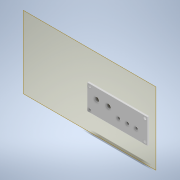
# Autodesk Inventor part: InterfacePlate
Saved by Autodesk Inventor 2022.2 (Build 262287000, 287)
## iProperties
Created: 2022-01-15
Part Number: InterfacePlate
Material: Generic
Document SubType Name: Modeling
Designer: siwat
Density: 1 g/cm^3
Appearance: Default
Author: siwat
Autodesk Inventor part; units mm, degrees
ref_plane "YZ Plane" through (0, 0, 0) normal (1, 0, 0) x (0, 1, 0)
ref_plane "XZ Plane" through (0, 0, 0) normal (0, 1, 0) x (-1, 0, 0)
ref_plane "XY Plane" through (0, 0, 0) normal (0, 0, 1) x (1, 0, 0)
ref_plane "Work Plane1" through (0, 0, 0) normal (0, 0, 1) x (1, 0, 0)
sketch "Sketch1" plane through (0, 0, 0) normal (0, 0, 1) x (1, 0, 0)
  line L0 (67.7271, 45.3897) -> (135.6749, 45.3897)
  line L1 (135.6749, 45.3897) -> (135.6749, 17.2701)
  line L2 (135.6749, 17.2701) -> (67.7271, 17.2701)
  line L3 (67.7271, 17.2701) -> (67.7271, 45.3897)
  circle A0 centre (70.3236, 42.7621) radius 1.5
  circle A1 centre (70.2655, 19.7679) radius 1.5
  circle A2 centre (132.8977, 19.6632) radius 1.5
  circle A3 centre (132.9442, 42.6673) radius 1.5
  point P0 (0, 0)
  dimension "d0" = 3
  dimension "d1" = 3
  dimension "d2" = 3
  dimension "d3" = 3
  constraints: 8 end point, 4 centre point, 2 parallel, 1 horizontal, 1 perpendicular
  measures "d0" diameter of A0
  measures "d1" diameter of A1
  measures "d2" diameter of A2
  measures "d3" diameter of A3
extrude "Extrusion1" add sketch "Sketch1" along normal blind 2
sketch "Sketch2" plane through (0, 0, 0) normal (0, 0, -1) x (-1, 0, 0)
  line L0 (-130.7904, 21.7727) -> (-72.4709, 21.7727)
  line L1 (-72.4709, 21.7727) -> (-72.4709, 40.605)
  line L2 (-72.4709, 40.605) -> (-130.7904, 40.605)
  line L3 (-130.7904, 40.605) -> (-130.7904, 21.7727)
  point P0 (0, 0)
  constraints: 8 end point, 2 parallel, 1 horizontal, 1 perpendicular
extrude "Extrusion2" add sketch "Sketch2" along normal blind 3
sketch "Sketch3" plane through (0, 0, -3) normal (0, 0, -1) x (-1, 0, 0)
  circle A0 centre (-123.1484, 27.6797) radius 1.75
  line L0 (-121.6186, 32.121) -> (-111.2555, 32.121)
  circle A1 centre (-113.1484, 27.6797) radius 1.75
  circle A2 centre (-103.1484, 27.6797) radius 1.75
  circle A3 centre (-91.5974, 33.7589) radius 2.5
  circle A4 centre (-78.3445, 33.7589) radius 2.5
  point P0 (0, 0)
  dimension "d8" = 3.5
  dimension "d11" = 10
  dimension "d16" = 5
  dimension "d17" = 5
  constraints: 5 centre point, 2 end point, 2 horizontal, 4 other
  measures "d8" diameter of A0
  measures "d11" distance of A0.centre A1.centre
  measures "d16" diameter of A3
  measures "d17" diameter of A4
extrude "Extrusion3" cut sketch "Sketch3" against normal up to surface (5 mm away)
sketch "Sketch4" plane through (0, 0, -3) normal (0, 0, -1) x (-1, 0, 0)
  line L0 (-126.3413, 33.4304) -> (-118.9387, 33.4304) construction
  line L1 (-118.9387, 33.4304) -> (-118.9387, 30.3319) construction
  line L2 (-118.9387, 30.3319) -> (-126.3413, 30.3319) construction
  line L3 (-126.3413, 30.3319) -> (-126.3413, 33.4304) construction
  line L4 (-116.3929, 33.3925) -> (-109.1583, 33.3925) construction
  line L5 (-109.1583, 33.3925) -> (-109.1583, 30.3319) construction
  line L6 (-109.1583, 30.3319) -> (-116.3929, 30.3319) construction
  line L7 (-116.3929, 30.3319) -> (-116.3929, 33.3925) construction
  line L8 (-107.7125, 33.476) -> (-98.1289, 33.476) construction
  line L9 (-98.1289, 33.476) -> (-98.1289, 30.3319) construction
  line L10 (-98.1289, 30.3319) -> (-107.7125, 30.3319) construction
  line L11 (-107.7125, 30.3319) -> (-107.7125, 33.476) construction
  line L12 (-95.4359, 29.1892) -> (-86.7439, 29.1892) construction
  line L13 (-86.7439, 29.1892) -> (-86.7439, 26.1412) construction
  line L14 (-86.7439, 26.1412) -> (-95.4359, 26.1412) construction
  line L15 (-95.4359, 26.1412) -> (-95.4359, 29.1892) construction
  line L16 (-80.7485, 29.2979) -> (-75.9197, 29.2979) construction
  line L17 (-75.9197, 29.2979) -> (-75.9197, 26.1412) construction
  line L18 (-75.9197, 26.1412) -> (-80.7485, 26.1412) construction
  line L19 (-80.7485, 26.1412) -> (-80.7485, 29.2979) construction
  line L20 (-123.6737, 30.3824) -> (-124.1998, 30.3824)
  line L21 (-124.1998, 30.3824) -> (-125.1631, 31.5952)
  line L22 (-125.1631, 31.5952) -> (-125.6275, 31.5952)
  line L23 (-125.6275, 31.5952) -> (-125.6275, 30.3824)
  line L24 (-125.6275, 30.3824) -> (-126.0326, 30.3824)
  line L25 (-126.0326, 30.3824) -> (-126.0326, 33.4304)
  line L26 (-126.0326, 33.4304) -> (-125.2471, 33.4304)
  spline S0 degree 2 poles (-125.2471, 33.4304) (-124.9853, 33.4304) (-124.6321, 33.3736) (-124.4715, 33.2699) knots 0 0 0 1 2 2 2
  spline S1 degree 2 poles (-124.4715, 33.2699) (-124.311, 33.1661) (-124.1257, 32.8426) (-124.1257, 32.603) knots 0 0 0 1 2 2 2
  spline S2 degree 2 poles (-124.1257, 32.603) (-124.1257, 32.2695) (-124.4666, 31.8175) (-124.758, 31.7088) knots 0 0 0 1 2 2 2
  line L27 (-124.758, 31.7088) -> (-123.6737, 30.3824)
  spline S3 degree 2 poles (-124.5481, 32.5709) (-124.5481, 32.7042) (-124.642, 32.9093) (-124.7408, 32.9759) knots 0 0 0 1 2 2 2
  spline S4 degree 2 poles (-124.7408, 32.9759) (-124.8272, 33.0328) (-125.0569, 33.0797) (-125.2249, 33.0797) knots 0 0 0 1 2 2 2
  line L28 (-125.2249, 33.0797) -> (-125.6275, 33.0797)
  line L29 (-125.6275, 33.0797) -> (-125.6275, 31.9336)
  line L30 (-125.6275, 31.9336) -> (-125.2718, 31.9336)
  spline S5 degree 2 poles (-125.2718, 31.9336) (-125.0964, 31.9336) (-124.8173, 31.9953) (-124.721, 32.0917) knots 0 0 0 1 2 2 2
  spline S6 degree 2 poles (-124.721, 32.0917) (-124.6321, 32.1757) (-124.5481, 32.4128) (-124.5481, 32.5709) knots 0 0 0 1 2 2 2
  line L31 (-123.4316, 30.3824) -> (-123.4316, 33.4304)
  line L32 (-123.4316, 33.4304) -> (-121.5248, 33.4304)
  line L33 (-121.5248, 33.4304) -> (-121.5248, 33.0698)
  line L34 (-121.5248, 33.0698) -> (-123.0266, 33.0698)
  line L35 (-123.0266, 33.0698) -> (-123.0266, 32.2349)
  line L36 (-123.0266, 32.2349) -> (-121.6261, 32.2349)
  line L37 (-121.6261, 32.2349) -> (-121.6261, 31.8743)
  line L38 (-121.6261, 31.8743) -> (-123.0266, 31.8743)
  line L39 (-123.0266, 31.8743) -> (-123.0266, 30.743)
  line L40 (-123.0266, 30.743) -> (-121.5248, 30.743)
  line L41 (-121.5248, 30.743) -> (-121.5248, 30.3824)
  line L42 (-121.5248, 30.3824) -> (-123.4316, 30.3824)
  line L43 (-120.3688, 30.3824) -> (-120.3688, 33.0698)
  line L44 (-120.3688, 33.0698) -> (-121.3914, 33.0698)
  line L45 (-121.3914, 33.0698) -> (-121.3914, 33.4304)
  line L46 (-121.3914, 33.4304) -> (-118.9412, 33.4304)
  line L47 (-118.9412, 33.4304) -> (-118.9412, 33.0698)
  line L48 (-118.9412, 33.0698) -> (-119.9637, 33.0698)
  line L49 (-119.9637, 33.0698) -> (-119.9637, 30.3824)
  line L50 (-119.9637, 30.3824) -> (-120.3688, 30.3824)
  line L51 (-116.0842, 30.3445) -> (-116.0842, 33.3925)
  line L52 (-116.0842, 33.3925) -> (-114.1773, 33.3925)
  line L53 (-114.1773, 33.3925) -> (-114.1773, 33.0319)
  line L54 (-114.1773, 33.0319) -> (-115.6791, 33.0319)
  line L55 (-115.6791, 33.0319) -> (-115.6791, 32.1971)
  line L56 (-115.6791, 32.1971) -> (-114.2786, 32.1971)
  line L57 (-114.2786, 32.1971) -> (-114.2786, 31.8364)
  line L58 (-114.2786, 31.8364) -> (-115.6791, 31.8364)
  line L59 (-115.6791, 31.8364) -> (-115.6791, 30.7052)
  line L60 (-115.6791, 30.7052) -> (-114.1773, 30.7052)
  line L61 (-114.1773, 30.7052) -> (-114.1773, 30.3445)
  line L62 (-114.1773, 30.3445) -> (-116.0842, 30.3445)
  line L63 (-111.6258, 30.3445) -> (-112.0902, 30.3445)
  line L64 (-112.0902, 30.3445) -> (-112.8312, 31.5598)
  line L65 (-112.8312, 31.5598) -> (-113.587, 30.3445)
  line L66 (-113.587, 30.3445) -> (-114.0242, 30.3445)
  line L67 (-114.0242, 30.3445) -> (-113.0535, 31.871)
  line L68 (-113.0535, 31.871) -> (-113.9946, 33.3925)
  line L69 (-113.9946, 33.3925) -> (-113.5302, 33.3925)
  line L70 (-113.5302, 33.3925) -> (-112.804, 32.1995)
  line L71 (-112.804, 32.1995) -> (-112.063, 33.3925)
  line L72 (-112.063, 33.3925) -> (-111.6258, 33.3925)
  line L73 (-111.6258, 33.3925) -> (-112.5792, 31.8908)
  line L74 (-112.5792, 31.8908) -> (-111.6258, 30.3445)
  line L75 (-110.5884, 30.3445) -> (-110.5884, 33.0319)
  line L76 (-110.5884, 33.0319) -> (-111.611, 33.0319)
  line L77 (-111.611, 33.0319) -> (-111.611, 33.3925)
  line L78 (-111.611, 33.3925) -> (-109.1607, 33.3925)
  line L79 (-109.1607, 33.3925) -> (-109.1607, 33.0319)
  line L80 (-109.1607, 33.0319) -> (-110.1833, 33.0319)
  line L81 (-110.1833, 33.0319) -> (-110.1833, 30.3445)
  line L82 (-110.1833, 30.3445) -> (-110.5884, 30.3445)
  line L83 (-106.6924, 30.3736) -> (-106.6924, 33.061)
  line L84 (-106.6924, 33.061) -> (-107.715, 33.061)
  line L85 (-107.715, 33.061) -> (-107.715, 33.4216)
  line L86 (-107.715, 33.4216) -> (-105.2647, 33.4216)
  line L87 (-105.2647, 33.4216) -> (-105.2647, 33.061)
  line L88 (-105.2647, 33.061) -> (-106.2873, 33.061)
  line L89 (-106.2873, 33.061) -> (-106.2873, 30.3736)
  line L90 (-106.2873, 30.3736) -> (-106.6924, 30.3736)
  line L91 (-104.956, 30.3736) -> (-104.956, 33.4216)
  line L92 (-104.956, 33.4216) -> (-103.0491, 33.4216)
  line L93 (-103.0491, 33.4216) -> (-103.0491, 33.061)
  line L94 (-103.0491, 33.061) -> (-104.5509, 33.061)
  line L95 (-104.5509, 33.061) -> (-104.5509, 32.2261)
  line L96 (-104.5509, 32.2261) -> (-103.1504, 32.2261)
  line L97 (-103.1504, 32.2261) -> (-103.1504, 31.8655)
  line L98 (-103.1504, 31.8655) -> (-104.5509, 31.8655)
  line L99 (-104.5509, 31.8655) -> (-104.5509, 30.7342)
  line L100 (-104.5509, 30.7342) -> (-103.0491, 30.7342)
  line L101 (-103.0491, 30.7342) -> (-103.0491, 30.3736)
  line L102 (-103.0491, 30.3736) -> (-104.956, 30.3736)
  spline S7 degree 2 poles (-101.7548, 30.3193) (-102.0858, 30.3193) (-102.5502, 30.4576) (-102.7552, 30.5564) knots 0 0 0 1 2 2 2
  line L103 (-102.7552, 30.5564) -> (-102.7552, 31.0652)
  line L104 (-102.7552, 31.0652) -> (-102.7256, 31.0652)
  spline S8 degree 2 poles (-102.7256, 31.0652) (-102.5255, 30.8775) (-102.0191, 30.67) (-101.7845, 30.67) knots 0 0 0 1 2 2 2
  spline S9 degree 2 poles (-101.7845, 30.67) (-101.4486, 30.67) (-101.1052, 30.9491) (-101.1052, 31.1788) knots 0 0 0 1 2 2 2
  spline S10 degree 2 poles (-101.1052, 31.1788) (-101.1052, 31.3616) (-101.2855, 31.5889) (-101.4807, 31.6457) knots 0 0 0 1 2 2 2
  spline S11 degree 2 poles (-101.4807, 31.6457) (-101.6215, 31.6852) (-101.8561, 31.7395) (-102.0315, 31.784) knots 0 0 0 1 2 2 2
  spline S12 degree 2 poles (-102.0315, 31.784) (-102.1896, 31.826) (-102.439, 31.952) (-102.5354, 32.0532) knots 0 0 0 1 2 2 2
  spline S13 degree 2 poles (-102.5354, 32.0532) (-102.6292, 32.1545) (-102.733, 32.4262) (-102.733, 32.604) knots 0 0 0 1 2 2 2
  spline S14 degree 2 poles (-102.733, 32.604) (-102.733, 32.9745) (-102.155, 33.476) (-101.7079, 33.476) knots 0 0 0 1 2 2 2
  spline S15 degree 2 poles (-101.7079, 33.476) (-101.451, 33.476) (-100.9966, 33.3747) (-100.8014, 33.2784) knots 0 0 0 1 2 2 2
  line L105 (-100.8014, 33.2784) -> (-100.8014, 32.7942)
  line L106 (-100.8014, 32.7942) -> (-100.8311, 32.7942)
  spline S16 degree 2 poles (-100.8311, 32.7942) (-100.9768, 32.9276) (-101.4313, 33.1252) (-101.6807, 33.1252) knots 0 0 0 1 2 2 2
  spline S17 degree 2 poles (-101.6807, 33.1252) (-101.9623, 33.1252) (-102.3106, 32.8609) (-102.3106, 32.646) knots 0 0 0 1 2 2 2
  spline S18 degree 2 poles (-102.3106, 32.646) (-102.3106, 32.4534) (-102.1056, 32.2237) (-101.9129, 32.1718) knots 0 0 0 1 2 2 2
  spline S19 degree 2 poles (-101.9129, 32.1718) (-101.7845, 32.1372) (-101.4115, 32.0483) (-101.288, 32.0112) knots 0 0 0 1 2 2 2
  spline S20 degree 2 poles (-101.288, 32.0112) (-100.9743, 31.9149) (-100.6829, 31.5271) (-100.6829, 31.2431) knots 0 0 0 1 2 2 2
  spline S21 degree 2 poles (-100.6829, 31.2431) (-100.6829, 31.0628) (-100.8286, 30.717) (-100.9595, 30.5959) knots 0 0 0 1 2 2 2
  spline S22 degree 2 poles (-100.9595, 30.5959) (-101.1052, 30.4625) (-101.4757, 30.3193) (-101.7548, 30.3193) knots 0 0 0 1 2 2 2
  line L107 (-99.559, 30.3736) -> (-99.559, 33.061)
  line L108 (-99.559, 33.061) -> (-100.5816, 33.061)
  line L109 (-100.5816, 33.061) -> (-100.5816, 33.4216)
  line L110 (-100.5816, 33.4216) -> (-98.1313, 33.4216)
  line L111 (-98.1313, 33.4216) -> (-98.1313, 33.061)
  line L112 (-98.1313, 33.061) -> (-99.1539, 33.061)
  line L113 (-99.1539, 33.061) -> (-99.1539, 30.3736)
  line L114 (-99.1539, 30.3736) -> (-99.559, 30.3736)
  spline S23 degree 2 poles (-93.2006, 28.2704) (-93.2006, 28.0728) (-93.3414, 27.7171) (-93.4673, 27.5936) knots 0 0 0 1 2 2 2
  spline S24 degree 2 poles (-93.4673, 27.5936) (-93.6254, 27.438) (-94.0527, 27.2775) (-94.3788, 27.2775) knots 0 0 0 1 2 2 2
  line L115 (-94.3788, 27.2775) -> (-94.7221, 27.2775)
  line L116 (-94.7221, 27.2775) -> (-94.7221, 26.1412)
  line L117 (-94.7221, 26.1412) -> (-95.1272, 26.1412)
  line L118 (-95.1272, 26.1412) -> (-95.1272, 29.1892)
  line L119 (-95.1272, 29.1892) -> (-94.3615, 29.1892)
  spline S25 degree 2 poles (-94.3615, 29.1892) (-94.0898, 29.1892) (-93.7094, 29.1003) (-93.5637, 28.9991) knots 0 0 0 1 2 2 2
  spline S26 degree 2 poles (-93.5637, 28.9991) (-93.3932, 28.883) (-93.2006, 28.5248) (-93.2006, 28.2704) knots 0 0 0 1 2 2 2
  spline S27 degree 2 poles (-93.6229, 28.2581) (-93.6229, 28.4161) (-93.7316, 28.6483) (-93.8428, 28.7224) knots 0 0 0 1 2 2 2
  spline S28 degree 2 poles (-93.8428, 28.7224) (-93.9391, 28.7866) (-94.196, 28.8385) (-94.3862, 28.8385) knots 0 0 0 1 2 2 2
  line L120 (-94.3862, 28.8385) -> (-94.7221, 28.8385)
  line L121 (-94.7221, 28.8385) -> (-94.7221, 27.6233)
  line L122 (-94.7221, 27.6233) -> (-94.4455, 27.6233)
  spline S29 degree 2 poles (-94.4455, 27.6233) (-94.1985, 27.6233) (-93.8946, 27.7023) (-93.7958, 27.806) knots 0 0 0 1 2 2 2
  spline S30 degree 2 poles (-93.7958, 27.806) (-93.7045, 27.8974) (-93.6229, 28.1123) (-93.6229, 28.2581) knots 0 0 0 1 2 2 2
  line L123 (-89.3992, 29.1892) -> (-90.1649, 26.1412)
  line L124 (-90.1649, 26.1412) -> (-90.6194, 26.1412)
  line L125 (-90.6194, 26.1412) -> (-91.2394, 28.6705)
  line L126 (-91.2394, 28.6705) -> (-91.8421, 26.1412)
  line L127 (-91.8421, 26.1412) -> (-92.2916, 26.1412)
  line L128 (-92.2916, 26.1412) -> (-93.0697, 29.1892)
  line L129 (-93.0697, 29.1892) -> (-92.6522, 29.1892)
  line L130 (-92.6522, 29.1892) -> (-92.0397, 26.6624)
  line L131 (-92.0397, 26.6624) -> (-91.432, 29.1892)
  line L132 (-91.432, 29.1892) -> (-91.0195, 29.1892)
  line L133 (-91.0195, 29.1892) -> (-90.407, 26.6328)
  line L134 (-90.407, 26.6328) -> (-89.7969, 29.1892)
  line L135 (-89.7969, 29.1892) -> (-89.3992, 29.1892)
  line L136 (-86.6773, 26.1412) -> (-87.2034, 26.1412)
  line L137 (-87.2034, 26.1412) -> (-88.1667, 27.354)
  line L138 (-88.1667, 27.354) -> (-88.631, 27.354)
  line L139 (-88.631, 27.354) -> (-88.631, 26.1412)
  line L140 (-88.631, 26.1412) -> (-89.0361, 26.1412)
  line L141 (-89.0361, 26.1412) -> (-89.0361, 29.1892)
  line L142 (-89.0361, 29.1892) -> (-88.2507, 29.1892)
  spline S31 degree 2 poles (-88.2507, 29.1892) (-87.9888, 29.1892) (-87.6356, 29.1324) (-87.4751, 29.0287) knots 0 0 0 1 2 2 2
  spline S32 degree 2 poles (-87.4751, 29.0287) (-87.3145, 28.925) (-87.1293, 28.6014) (-87.1293, 28.3618) knots 0 0 0 1 2 2 2
  spline S33 degree 2 poles (-87.1293, 28.3618) (-87.1293, 28.0283) (-87.4701, 27.5763) (-87.7616, 27.4676) knots 0 0 0 1 2 2 2
  line L143 (-87.7616, 27.4676) -> (-86.6773, 26.1412)
  spline S34 degree 2 poles (-87.5516, 28.3297) (-87.5516, 28.4631) (-87.6455, 28.6681) (-87.7443, 28.7348) knots 0 0 0 1 2 2 2
  spline S35 degree 2 poles (-87.7443, 28.7348) (-87.8308, 28.7916) (-88.0605, 28.8385) (-88.2284, 28.8385) knots 0 0 0 1 2 2 2
  line L144 (-88.2284, 28.8385) -> (-88.631, 28.8385)
  line L145 (-88.631, 28.8385) -> (-88.631, 27.6924)
  line L146 (-88.631, 27.6924) -> (-88.2754, 27.6924)
  spline S36 degree 2 poles (-88.2754, 27.6924) (-88.1, 27.6924) (-87.8209, 27.7542) (-87.7245, 27.8505) knots 0 0 0 1 2 2 2
  spline S37 degree 2 poles (-87.7245, 27.8505) (-87.6356, 27.9345) (-87.5516, 28.1716) (-87.5516, 28.3297) knots 0 0 0 1 2 2 2
  spline S38 degree 2 poles (-78.5132, 28.3247) (-78.5132, 28.1271) (-78.654, 27.7715) (-78.7799, 27.648) knots 0 0 0 1 2 2 2
  spline S39 degree 2 poles (-78.7799, 27.648) (-78.938, 27.4923) (-79.3653, 27.3318) (-79.6914, 27.3318) knots 0 0 0 1 2 2 2
  line L147 (-79.6914, 27.3318) -> (-80.0347, 27.3318)
  line L148 (-80.0347, 27.3318) -> (-80.0347, 26.1956)
  line L149 (-80.0347, 26.1956) -> (-80.4398, 26.1956)
  line L150 (-80.4398, 26.1956) -> (-80.4398, 29.2436)
  line L151 (-80.4398, 29.2436) -> (-79.6741, 29.2436)
  spline S40 degree 2 poles (-79.6741, 29.2436) (-79.4024, 29.2436) (-79.022, 29.1547) (-78.8763, 29.0534) knots 0 0 0 1 2 2 2
  spline S41 degree 2 poles (-78.8763, 29.0534) (-78.7058, 28.9373) (-78.5132, 28.5792) (-78.5132, 28.3247) knots 0 0 0 1 2 2 2
  spline S42 degree 2 poles (-78.9356, 28.3124) (-78.9356, 28.4705) (-79.0442, 28.7027) (-79.1554, 28.7768) knots 0 0 0 1 2 2 2
  spline S43 degree 2 poles (-79.1554, 28.7768) (-79.2517, 28.841) (-79.5086, 28.8928) (-79.6988, 28.8928) knots 0 0 0 1 2 2 2
  line L152 (-79.6988, 28.8928) -> (-80.0347, 28.8928)
  line L153 (-80.0347, 28.8928) -> (-80.0347, 27.6776)
  line L154 (-80.0347, 27.6776) -> (-79.7581, 27.6776)
  spline S44 degree 2 poles (-79.7581, 27.6776) (-79.5111, 27.6776) (-79.2073, 27.7566) (-79.1085, 27.8604) knots 0 0 0 1 2 2 2
  spline S45 degree 2 poles (-79.1085, 27.8604) (-79.0171, 27.9518) (-78.9356, 28.1667) (-78.9356, 28.3124) knots 0 0 0 1 2 2 2
  spline S46 degree 2 poles (-76.9373, 26.1412) (-77.2337, 26.1412) (-77.7351, 26.3413) (-77.9179, 26.5414) knots 0 0 0 1 2 2 2
  spline S47 degree 2 poles (-77.9179, 26.5414) (-78.1007, 26.739) (-78.3008, 27.3318) (-78.3008, 27.7171) knots 0 0 0 1 2 2 2
  spline S48 degree 2 poles (-78.3008, 27.7171) (-78.3008, 28.1) (-78.1056, 28.6681) (-77.9204, 28.878) knots 0 0 0 1 2 2 2
  spline S49 degree 2 poles (-77.9204, 28.878) (-77.7376, 29.083) (-77.2387, 29.2979) (-76.9299, 29.2979) knots 0 0 0 1 2 2 2
  spline S50 degree 2 poles (-76.9299, 29.2979) (-76.7768, 29.2979) (-76.5075, 29.2535) (-76.3939, 29.2189) knots 0 0 0 1 2 2 2
  spline S51 degree 2 poles (-76.3939, 29.2189) (-76.2951, 29.1868) (-76.0901, 29.0954) (-75.9888, 29.041) knots 0 0 0 1 2 2 2
  line L155 (-75.9888, 29.041) -> (-75.9888, 28.552)
  line L156 (-75.9888, 28.552) -> (-76.0209, 28.552)
  spline S52 degree 2 poles (-76.0209, 28.552) (-76.0753, 28.6014) (-76.2432, 28.7397) (-76.3643, 28.8064) knots 0 0 0 1 2 2 2
  spline S53 degree 2 poles (-76.3643, 28.8064) (-76.4804, 28.8706) (-76.7545, 28.9521) (-76.9324, 28.9521) knots 0 0 0 1 2 2 2
  spline S54 degree 2 poles (-76.9324, 28.9521) (-77.1275, 28.9521) (-77.4758, 28.7916) (-77.6067, 28.6384) knots 0 0 0 1 2 2 2
  spline S55 degree 2 poles (-77.6067, 28.6384) (-77.7351, 28.4828) (-77.8784, 28.0111) (-77.8784, 27.7171) knots 0 0 0 1 2 2 2
  spline S56 degree 2 poles (-77.8784, 27.7171) (-77.8784, 27.4034) (-77.7277, 26.9514) (-77.5968, 26.7958) knots 0 0 0 1 2 2 2
  spline S57 degree 2 poles (-77.5968, 26.7958) (-77.4684, 26.6451) (-77.125, 26.492) (-76.9324, 26.492) knots 0 0 0 1 2 2 2
  spline S58 degree 2 poles (-76.9324, 26.492) (-76.757, 26.492) (-76.4581, 26.5784) (-76.342, 26.6427) knots 0 0 0 1 2 2 2
  spline S59 degree 2 poles (-76.342, 26.6427) (-76.2309, 26.7069) (-76.0654, 26.8403) (-76.0185, 26.8872) knots 0 0 0 1 2 2 2
  line L157 (-76.0185, 26.8872) -> (-75.9888, 26.8872)
  line L158 (-75.9888, 26.8872) -> (-75.9888, 26.4031)
  spline S60 degree 2 poles (-75.9888, 26.4031) (-76.0901, 26.3561) (-76.2679, 26.2697) (-76.3939, 26.2302) knots 0 0 0 1 2 2 2
  spline S61 degree 2 poles (-76.3939, 26.2302) (-76.5273, 26.1857) (-76.7545, 26.1412) (-76.9373, 26.1412) knots 0 0 0 1 2 2 2
  point P0 (0, 0)
  constraints: 3 collinear, 10 other
extrude "Extrusion4" cut sketch "Sketch4" against normal blind 1.5
body "Solid1"
